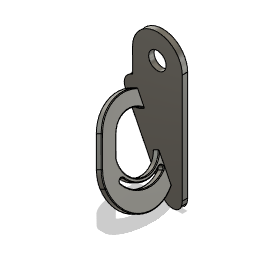
Dispositif antichute (Autodesk Fusion 360 design; units mm, degrees)
Autodesk Fusion 360 part; units mm, degrees
sketch "Sketch1" plane through (0, 0, 0) normal (0, 0, 1) x (1, 0, 0)
  line L0 (34.1353, 28.7505) -> (76.2882, 28.7505) construction
  line L1 (55.191, 53.2671) -> (55.191, 4.3332) construction
  circle A0 centre (55.191, 28.8002) radius 18.4477
  line L2 (36.7433, 28.7505) -> (36.7911, 11.0227)
  line L3 (73.6386, 28.7505) -> (73.6386, -52.3324)
  line L4 (73.6386, -62.6389) -> (36.7911, 11.0227)
  line L5 (69.1669, -64.8758) -> (32.3194, 8.7858)
  line L6 (36.7911, 11.0227) -> (32.3194, 8.7858)
  line L7 (73.6386, -62.6389) -> (69.1669, -64.8758)
  line L8 (71.7392, -58.8419) -> (72.0517, -58.2963)
  arc A1 (72.0517, -58.2963) -> (73.6386, -52.3324) centre (61.6386, -52.3324) ccw
  dimension "d1" = 5
  dimension "d2" = 12
  constraint horizontal L0
  constraint vertical L1
  constraint midpoint L1 A0.centre
  constraint coincident A0 L2.start
  constraint coincident L0 L2.start
  constraint tangent A0 L2
  constraint coincident A0 L3.start
  constraint coincident L0 L3.start
  constraint perpendicular L0 L3
  constraint coincident L4 L8.start
  constraint tangent L8 A1
  constraint tangent L3 A1
  measures "d2" radius of A1
extrude "Extrude1" add sketch "Sketch1" along normal blind 4
sketch "Sketch2" plane through (0, 0, 4) normal (0, 0, 1) x (1, 0, 0)
  line L0 (73.6386, -62.6389) -> (71.7392, -58.8419)
  line L1 (71.7392, -58.8419) -> (72.0517, -58.2963)
  arc A0 (72.0517, -58.2963) -> (73.6386, -52.3324) centre (61.6386, -52.3324) ccw
  line L2 (73.6386, -52.3324) -> (73.6386, 28.7505)
  arc A1 (73.6386, 28.7505) -> (36.7433, 28.7505) centre (55.191, 28.8002) ccw
  line L3 (36.7433, 28.7505) -> (36.7911, 11.0227)
  line L4 (36.7911, 11.0227) -> (32.3194, 8.7858)
  line L5 (32.3194, 8.7858) -> (69.1669, -64.8758)
  line L6 (69.1669, -64.8758) -> (73.6386, -62.6389)
  line L7 (73.6386, -62.6389) -> (69.1669, -64.8758)
  line L8 (69.1669, -64.8758) -> (32.3194, 8.7858)
  line L9 (32.3194, 8.7858) -> (36.7911, 11.0227)
  line L10 (36.7911, 11.0227) -> (73.6386, -62.6389)
  constraint perpendicular L7 L8
  constraint parallel L7 L9
  constraint parallel L8 L10
  constraint coincident L5.end L6.start
  constraint perpendicular L5 L7
  constraint coincident L0.start L6.end
extrude "Extrude2" add sketch "Sketch2" along normal blind 42 contours L0 L4 L5 L6 L7 L8 L9 L10
sketch "Sketch3" plane through (33.8378, 16.9266, 0) normal (0.894346, 0.447376, 0) x (0, 0, -1)
  line L0 (0, -88.965) -> (0, -84.7194)
  line L1 (0, -84.7194) -> (-4, -84.7194)
  line L2 (-4, -84.7194) -> (-4, -6.6014)
  line L3 (-4, -6.6014) -> (-46, -6.6014)
  line L4 (-46, -6.6014) -> (-46, -88.965)
  line L5 (-46, -88.965) -> (0, -88.965)
sketch "Sketch4" plane through (33.8378, 16.9266, 0) normal (0.894346, 0.447376, 0) x (0, 0, -1)
  line L0 (-26.7558, -30.7677) -> (-32.1249, -42.8155)
  line L1 (-35.8898, -26.6971) -> (-41.2589, -38.7449)
  arc A0 (-32.1249, -42.8155) -> (-4, -50.1388) centre (-17.544, -44.4859) ccw
  line L2 (-4, -84.7194) -> (-4, -6.6014)
  line L3 (-4, -79.7475) -> (-4, -7.2313)
  line L4 (-4, -14.4741) -> (16.8302, -14.4741)
  arc A1 (-4, -14.4741) -> (-35.8898, -26.6971) centre (-13.8352, -36.5258) ccw
  arc A2 (-4, -26.3589) -> (-26.7558, -30.7677) centre (-13.8352, -36.5258) ccw
  arc A3 (-31.8855, -54.1157) -> (-7.7112, -58.2415) centre (-17.7652, -44.2659) ccw
  arc A4 (-34.7561, -56.1181) -> (-5.6672, -61.0826) centre (-17.7652, -44.2659) ccw
  arc A5 (-5.6672, -61.0826) -> (-7.7112, -58.2415) centre (-6.6892, -59.662) ccw
  arc A6 (-31.8855, -54.1157) -> (-34.7561, -56.1181) centre (-33.3208, -55.1169) ccw
  line L5 (-41.2589, -38.7449) -> (-43.5757, -43.9434)
  arc A7 (-45.4319, -54.365) -> (-4, -71.1372) centre (-20.651, -52.7097) ccw
  arc A8 (-43.5757, -43.9434) -> (-45.4319, -54.365) centre (-23.4808, -52.8987) ccw
  line L6 (-4, -6.6014) -> (-46, -6.6014)
  line L7 (-46, -6.6014) -> (-46, -88.965)
  line L8 (-46, -88.965) -> (0, -88.965)
  line L9 (0, -88.965) -> (0, -84.7194)
  line L10 (-4, -6.6014) -> (-4, -84.7194)
  line L11 (0, -84.7194) -> (-4, -84.7194)
  dimension "d9" = 3.5
  dimension "d10" = 22
  constraint coincident A0.end L2
  constraint coincident L2 L4.start
  constraint perpendicular L2 L4
  constraint tangent L1 A1
  constraint concentric A1 A2
  constraint coincident L2 A2.start
  constraint parallel L0 L1
  constraint tangent A3 A6
  constraint tangent A4 A5
  constraint parallel L1 L5
  constraint coincident L2 A7.end
  constraint tangent A7 A8
  constraint tangent L5 A8
  measures "d10" radius of A8
extrude "Extrude3" cut sketch "Sketch4" against normal through all contours L0 A0 L2 L3 A2 L10 | L1 L2 L3 A1 L5 A7 A8 L6 L7 L8 L9 L10 L11 | A3 A4 A5 A6
sketch "Sketch5" plane through (29.3661, 14.6897, 0) normal (-0.894346, -0.447376, 0) x (0, 0, 1)
  line L0 (0, -84.7194) -> (4, -84.7194)
  line L1 (4, -84.7194) -> (4, -71.1372)
  arc A0 (4, -71.1372) -> (45.4319, -54.365) centre (20.651, -52.7097) ccw
  arc A1 (45.4319, -54.365) -> (43.5757, -43.9434) centre (23.4808, -52.8987) ccw
  line L2 (43.5757, -43.9434) -> (35.8898, -26.6971)
  arc A2 (35.8898, -26.6971) -> (4, -14.4741) centre (13.8352, -36.5258) ccw
  line L3 (4, -14.4741) -> (4, -6.6014)
  line L4 (4, -6.6014) -> (0, -6.6014)
  line L5 (0, -6.6014) -> (0, -84.7194)
  arc A3 (7.7112, -58.2415) -> (31.8855, -54.1157) centre (17.7652, -44.2659) ccw
  arc A4 (34.7561, -56.1181) -> (31.8855, -54.1157) centre (33.3208, -55.1169) ccw
  arc A5 (5.6672, -61.0826) -> (34.7561, -56.1181) centre (17.7652, -44.2659) ccw
  arc A6 (7.7112, -58.2415) -> (5.6672, -61.0826) centre (6.6892, -59.662) ccw
  line L6 (4, -50.1388) -> (4, -26.3589)
  arc A7 (26.7558, -30.7677) -> (4, -26.3589) centre (13.8352, -36.5258) ccw
  line L7 (26.7558, -30.7677) -> (32.1249, -42.8155)
  arc A8 (4, -50.1388) -> (32.1249, -42.8155) centre (17.544, -44.4859) ccw
  line L8 (4, -84.7194) -> (0, -84.7194)
  line L9 (0, -84.7194) -> (0, -6.6014)
  line L10 (0, -6.6014) -> (4, -6.6014)
  line L11 (4, -6.6014) -> (4, -84.7194)
  constraint horizontal L8
  constraint vertical L9
  constraint horizontal L10
  constraint vertical L11
  constraint coincident L4.end L5.start
  constraint coincident L0.end L1.start
extrude "Extrude4" add sketch "Sketch5" along normal blind 5 contours L0 L1 L3 L4 L5 L6 L8 L9 L10 L11
sketch "Sketch6" plane through (0, 0, 4) normal (0, 0, 1) x (1, 0, 0)
  line L0 (62.7958, -63.3156) -> (71.7392, -58.8419)
  line L1 (71.7392, -58.8419) -> (72.0517, -58.2963)
  arc A0 (72.0517, -58.2963) -> (73.6386, -52.3324) centre (61.6386, -52.3324) ccw
  line L2 (73.6386, -52.3324) -> (73.6386, 28.7505)
  arc A1 (73.6386, 28.7505) -> (36.7433, 28.7505) centre (55.191, 28.8002) ccw
  line L3 (36.7433, 28.7505) -> (36.7911, 11.0227)
  line L4 (36.7911, 11.0227) -> (27.8476, 6.5489)
  line L5 (27.8476, 6.5489) -> (62.7958, -63.3156)
  line L6 (61.1911, -48.9315) -> (51.797, -30.1517)
  line L7 (51.797, -30.1517) -> (56.2687, -27.9148)
  line L8 (56.2687, -27.9148) -> (65.6629, -46.6946)
  line L9 (65.6629, -46.6946) -> (61.1911, -48.9315)
  line L10 (41.1584, -8.8842) -> (35.8414, 1.7449)
  line L11 (35.8414, 1.7449) -> (40.3131, 3.9818)
  line L12 (40.3131, 3.9818) -> (45.6301, -6.6473)
  line L13 (45.6301, -6.6473) -> (41.1584, -8.8842)
  arc A2 (73.6386, 28.7505) -> (36.7433, 28.7505) centre (55.191, 28.8002) ccw
  circle A3 centre (55.191, 28.8002) radius 6.5
  dimension "d14" = 13
  constraint concentric A1 A3
  measures "d14" diameter of A3
extrude "Extrude5" cut sketch "Sketch6" against normal through all contours A3
fillet "Fillet1" radius 8 2 edges at (27.8476, 6.5489, 2) (62.7958, -63.3156, 2)
fillet "Fillet2" radius 6.5 1 edges at (71.7392, -58.8419, 2)
fillet "Fillet3" radius 0.5 8 edges at (40.0919, 4.424, 22.4769) (49.6392, -14.6619, 39.7327) (55.7775, -26.9329, 45.1399) (67.718, -50.8031, 29.9704) (63.2463, -53.04, 29.9704) (51.3058, -29.1698, 45.1399) (45.1675, -16.8988, 39.7327) (35.6202, 2.1871, 22.4769)
fillet "Fillet4" radius 0.5 14 edges at (50.2975, -15.9778, 29.4404) (43.9657, -3.32, 16.5258) (39.494, -5.5569, 16.5258) (45.8257, -18.2147, 29.4404) (55.622, -37.7983, 21.2422) (60.0937, -35.5614, 21.2422) (61.2337, -37.8403, 20.6616) (60.072, -35.5179, 5.2686) (62.7772, -40.9259, 21.2504) (57.8537, -31.0833, 34.322) (58.3055, -43.1628, 21.2504) (55.6002, -37.7548, 5.2686) (56.762, -40.0772, 20.6616) (53.3819, -33.3202, 34.322)
